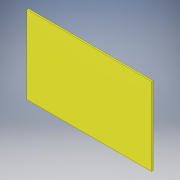
# Autodesk Inventor part: 電控板
Saved by Autodesk Inventor 2019 (Build 230136000, 136)
## iProperties
Created: 2018-08-23
Part Number: 電控板
Material: 鐵、灰色
Document SubType Name: Modeling
Designer: elecjack
Density: 7.15 g/cm^3
Appearance: 黃
Author: elecjack
Autodesk Inventor part; units mm, degrees
ref_plane "YZ Plane" through (0, 0, 0) normal (1, 0, 0) x (0, 1, 0)
ref_plane "XZ Plane" through (0, 0, 0) normal (0, 1, 0) x (-1, 0, 0)
ref_plane "XY Plane" through (0, 0, 0) normal (0, 0, 1) x (1, 0, 0)
sketch "草圖1" plane through (0, 0, 0) normal (0, 0, 1) x (1, 0, 0)
  line L0 (-400, 250) -> (400, 250)
  line L1 (400, 250) -> (400, -250)
  line L2 (400, -250) -> (-400, -250)
  line L3 (-400, -250) -> (-400, 250)
  point P0 (0, 0)
  dimension "d0" = 800
  dimension "d1" = 400
  dimension "d2" = 500
  dimension "d3" = 250
  constraints: 8 end point, 2 parallel, 1 horizontal, 1 perpendicular
  measures "d0" distance between parallel lines of L1 L3
  measures "d1" distance from line of point (0, 0) L3
  measures "d2" distance between parallel lines of L0 L2
  measures "d3" distance from line of point (0, 0) L2
extrude "擠出1" add sketch "草圖1" along normal blind 10
